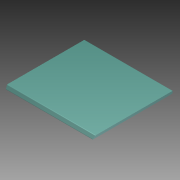
# Autodesk Inventor part: Tapa batería
Saved by Autodesk Inventor 2014 (Build 180170000, 170)
## iProperties
Created: 2017-06-20
Part Number: Tapa batería
Material: Generic
Document SubType Name: Modeling
Designer: resaj
Density: 1 g/cm^3
Appearance: Indoor Pool
Author: resaj
Autodesk Inventor part; units mm, degrees
ref_plane "YZ Plane" through (0, 0, 0) normal (1, 0, 0) x (0, 1, 0)
ref_plane "XZ Plane" through (0, 0, 0) normal (0, 1, 0) x (-1, 0, 0)
sketch "Sketch1" plane through (0, 0, 0) normal (0, 1, 0) x (-1, 0, 0)
  line L0 (0, 0) -> (62.5, 0)
  line L1 (62.5, 0) -> (62.5, 56.8)
  line L2 (62.5, 56.8) -> (0, 56.8)
  line L3 (0, 56.8) -> (0, 0)
  dimension "d7" = 62.5
  dimension "d8" = 56.8
  constraints: 8 end point, 2 parallel, 1 horizontal, 1 perpendicular
  measures "d7" distance of L1.end L2.end
  measures "d8" distance of L0.end L1.end
extrude "Extrusion1" add sketch "Sketch1" along normal blind 3
sketch "Sketch2" plane through (0, 0, 56.8) normal (1, 0, 0) x (0, 0, -1)
  line L0 (56.8, 0) -> (56.8, 3) projected
  line L1 (0, 3) -> (56.8, 3) projected
  line L2 (0, 0) -> (0, 3) projected
  line L3 (0, 0) -> (1, 3)
  line L4 (56.8, 0) -> (55.8, 3)
  dimension "d2" = 1
  dimension "d3" = 1
  constraints: 4 end point, 2 point on line
  measures "d2" distance of L1.start L3.end
  measures "d3" distance of L0.end L4.end
extrude "Extrusion2" cut sketch "Sketch2" against normal through all
fillet "Fillet1" radius 0.5 4 edges at (-31.25, 3, 55.8) (-31.25, 0, 56.8) (-31.25, 3, 1) (-31.25, 0, 0)
ref_plane "Work Plane1" through (0, 3, 28.4) normal (0, 0, -1) x (-1, 0, 0)
sketch "Sketch3" plane through (0, 3, 28.4) normal (0, 0, -1) x (-1, 0, 0)
  line L0 (62.5, 0) -> (62.5, -3) projected
  line L1 (62.5, -3) -> (0, -3) projected
  line L2 (0, -3) -> (0, 0) projected
  line L3 (0, 0) -> (62.5, 0) projected
  line L4 (0, 0) -> (1.3849, -3)
  dimension "d12" = 65.22
  constraints: 2 end point, 1 point on line
  measures "d12" angle of L3 L4
extrude "Extrusion3" cut sketch "Sketch3" along normal through all both and the other way through all contours L4 L1 L2
body "Solid1"
